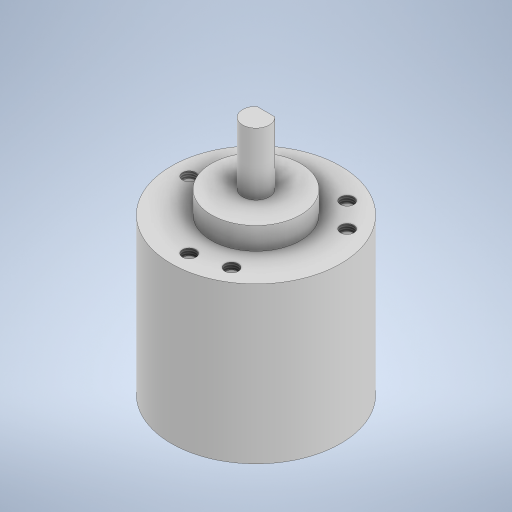
# Autodesk Inventor part: rotary_encoder
Saved by Autodesk Inventor 2023 (Build 270158000, 158)
## iProperties
Created: 2024-02-27
Part Number: rotary_encoder
Material: 常规
Document SubType Name: Modeling
Designer: Nitrene.P.L
Density: 1 g/cm^3
Appearance: 默认
Author: Nitrene.P.L
Autodesk Inventor part; units mm, degrees
ref_plane "YZ Plane" through (0, 0, 0) normal (1, 0, 0) x (0, 1, 0)
ref_plane "XZ Plane" through (0, 0, 0) normal (0, 1, 0) x (-1, 0, 0)
ref_plane "XY Plane" through (0, 0, 0) normal (0, 0, 1) x (1, 0, 0)
sketch "草图1" plane through (0, 0, 0) normal (0, 1, 0) x (-1, 0, 0)
  circle A0 centre (0, 0) radius 19
  circle A1 centre (0, 0) radius 10
  dimension "d0" = 38
  dimension "d1" = 20
  constraints: 2 centre point, 2 coincident
  measures "d0" diameter of A0
  measures "d1" diameter of A1
extrude "拉伸1" add sketch "草图1" against normal blind 35 contours A0 | A1
sketch "草图2" plane through (0, 0, 0) normal (0, 1, 0) x (1, 0, 0)
  circle A0 centre (0, 0) radius 10
  circle A1 centre (0, 0) radius 15
  circle A2 centre (-15, 0) radius 1.5
  circle A3 centre (7.5, -12.9904) radius 1.5
  circle A4 centre (7.5, 12.9904) radius 1.5
  line L0 (0, 0) -> (-12.9904, 7.5)
  line L1 (0, 0) -> (15, 0) construction
  circle A5 centre (-12.9904, 7.5) radius 1.5
  circle A6 centre (0, -15) radius 1.5
  circle A7 centre (12.9904, 7.5) radius 1.5
  dimension "d4" = 20
  dimension "d5" = 30
  dimension "d6" = 3
  dimension "d9" = 360
  dimension "d11" = 150
  dimension "d12" = 3
  dimension "d15" = 360
  constraints: 8 centre point, 4 end point, 3 coincident, 2 point on circle, 1 equal length, 1 horizontal, 14 other
  measures "d4" diameter of A0
  measures "d5" diameter of A1
  measures "d6" diameter of A2
  measures "d11" angle of L1 L0
  measures "d12" diameter of A5
extrude "拉伸2" cut sketch "草图2" against normal blind 1.5 contours A5 A1 L0 | L0 A1 A5 | A1 A5 | A2 A1 | A1 A2 | A4 A1 | A1 A4 | A6 A1 | A1 A6 | A7 A1 | A1 A7 | A3 A1 | A1 A3
sketch "草图3" plane through (0, 0, 0) normal (0, 1, 0) x (1, 0, 0)
  circle A0 centre (0, 0) radius 10
  dimension "d19" = 20
  constraints: 1 centre point, 1 coincident
  measures "d19" diameter of A0
extrude "拉伸3" add sketch "草图3" along normal blind 5
sketch "草图4" plane through (0, 5, 0) normal (0, 1, 0) x (1, 0, 0)
  circle A0 centre (0, 0) radius 3
  dimension "d22" = 6
  constraints: 1 centre point, 1 coincident
  measures "d22" diameter of A0
extrude "拉伸4" add sketch "草图4" along normal blind 14
sketch "草图5" plane through (0, 19, 0) normal (0, 1, 0) x (1, 0, 0)
  circle A0 centre (0, 0) radius 3 projected
  line L0 (0, -3) -> (0, 2.2)
  line L1 (0, 2.2) -> (-2.0396, 2.2)
  line L2 (0, 2.2) -> (2.0396, 2.2)
  dimension "d25" = 5.2
  constraints: 6 end point, 3 point on circle, 1 horizontal, 1 point on line, 1 vertical
  measures "d25" distance of L0.start L0.end
extrude "拉伸5" cut sketch "草图5" against normal blind 10 contours L2 L1 A0
thread "螺纹1" size "M3x0.5" class "6H" standard "ANSI Metric M Profile" length 1.5
thread "螺纹2" size "M3x0.5" class "6H" standard "ANSI Metric M Profile" length 1.5
thread "螺纹3" size "M3x0.5" class "6H" standard "ANSI Metric M Profile" length 1.5
thread "螺纹4" size "M3x0.5" class "6H" standard "ANSI Metric M Profile" length 1.5
thread "螺纹5" size "M3x0.5" class "6H" standard "ANSI Metric M Profile" length 1.5
thread "螺纹6" size "M3x0.5" class "6H" standard "ANSI Metric M Profile" length 1.5
